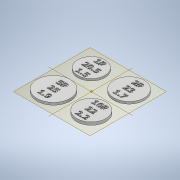
# Autodesk Inventor part: Монеты
Saved by Autodesk Inventor 2020 (Build 240168000, 168)
## iProperties
Created: 2019-12-21
Part Number: Монеты
Material: Типовые
Document SubType Name: Modeling
Designer: Css38
Density: 1 g/cm^3
Appearance: По умолчанию
Author: Css38
Autodesk Inventor part; units mm, degrees
ref_plane "YZ Plane" through (0, 0, 0) normal (1, 0, 0) x (0, 1, 0)
ref_plane "XZ Plane" through (0, 0, 0) normal (0, 1, 0) x (-1, 0, 0)
sketch "Эскиз1" plane through (0, 0, 0) normal (0, 0, 1) x (1, 0, 0)
  circle A0 centre (-14.2806, 14.2806) radius 10.25
  circle A1 centre (14.2806, 14.2806) radius 11.5
  circle A2 centre (-14.2806, -14.2806) radius 12.5
  circle A3 centre (14.2806, -14.2806) radius 11
  line L0 (-37.2928, 0) -> (36.2928, 0) construction
  line L1 (-14.2806, -14.2806) -> (-14.2806, 0) construction
  line L2 (-14.2806, -14.2806) -> (0, -14.2806) construction
  line L3 (14.2806, -14.2806) -> (0, -14.2806) construction
  line L4 (14.2806, -14.2806) -> (14.2806, 0) construction
  line L5 (14.2806, 14.2806) -> (14.2806, 0) construction
  line L6 (14.2806, 14.2806) -> (0, 14.2806) construction
  line L7 (0, 14.2806) -> (-14.2806, 14.2806) construction
  line L8 (-14.2806, 14.2806) -> (-14.2806, 0) construction
  line L9 (0, -37.2928) -> (0, 36.2928) construction
  point P0 (0, 0)
  dimension "d0" = 20.5
  dimension "d1" = 23
  dimension "d2" = 25
  dimension "d3" = 22
  constraints: 16 end point, 8 perpendicular, 4 centre point, 3 point on line, 2 collinear, 2 horizontal, 2 horizontal alignment, 2 vertical alignment
  measures "d0" diameter of A0
  measures "d1" diameter of A1
  measures "d2" diameter of A2
  measures "d3" diameter of A3
extrude "Выдавливание1" add sketch "Эскиз1" along normal blind 1.5 contours A0
extrude "Выдавливание2" add sketch "Эскиз1" along normal blind 1.7 contours A1
extrude "Выдавливание3" add sketch "Эскиз1" along normal blind 1.8 contours A2
extrude "Выдавливание4" add sketch "Эскиз1" along normal blind 2.2 contours A3
sketch "Эскиз2" plane through (-14.2806, 14.2806, 1.5) normal (0, 0, 1) x (1, 0, 0)
  line L0 (-10.25, 10.25) -> (10.25, 10.25) construction
  line L1 (10.25, 10.25) -> (10.25, -10.25) construction
  line L2 (10.25, -10.25) -> (-10.25, -10.25) construction
  line L3 (-10.25, -10.25) -> (-10.25, 10.25) construction
  circle A0 centre (0, 0) radius 10.25 construction
  line L4 (-0.3371, 4.6232) -> (-2.9789, 4.6232)
  line L5 (-2.9789, 4.6232) -> (-2.9789, 5.3201)
  line L6 (-2.9789, 5.3201) -> (-2.1361, 5.3201)
  line L7 (-2.1361, 5.3201) -> (-2.1361, 7.4368)
  line L8 (-2.1361, 7.4368) -> (-2.9789, 7.4368)
  line L9 (-2.9789, 7.4368) -> (-2.9789, 8.0883)
  spline S0 degree 2 poles (-2.9789, 8.0883) (-2.7942, 8.0883) (-2.4279, 8.1369) (-2.3177, 8.1888) knots 0 0 0 1 2 2 2
  spline S1 degree 2 poles (-2.3177, 8.1888) (-2.1912, 8.2536) (-2.0486, 8.4708) (-2.0357, 8.6329) knots 0 0 0 1 2 2 2
  line L10 (-2.0357, 8.6329) -> (-1.1605, 8.6329)
  line L11 (-1.1605, 8.6329) -> (-1.1605, 5.3201)
  line L12 (-1.1605, 5.3201) -> (-0.3371, 5.3201)
  line L13 (-0.3371, 5.3201) -> (-0.3371, 4.6232)
  line L14 (2.4084, 5.6929) -> (2.4084, 5.1224)
  line L15 (2.4084, 5.1224) -> (1.3323, 5.1224)
  line L16 (1.3323, 5.1224) -> (1.3323, 4.6232)
  line L17 (1.3323, 4.6232) -> (0.3339, 4.6232)
  line L18 (0.3339, 4.6232) -> (0.3339, 5.1224)
  line L19 (0.3339, 5.1224) -> (0.0583, 5.1224)
  line L20 (0.0583, 5.1224) -> (0.0583, 5.6929)
  line L21 (0.0583, 5.6929) -> (0.3339, 5.6929)
  line L22 (0.3339, 5.6929) -> (0.3339, 6.0916)
  line L23 (0.3339, 6.0916) -> (0.0583, 6.0916)
  line L24 (0.0583, 6.0916) -> (0.0583, 6.8112)
  line L25 (0.0583, 6.8112) -> (0.3339, 6.8112)
  line L26 (0.3339, 6.8112) -> (0.3339, 8.6232)
  line L27 (0.3339, 8.6232) -> (1.8606, 8.6232)
  spline S2 degree 2 poles (1.8606, 8.6232) (2.1783, 8.6232) (2.7358, 8.4903) (3.1475, 8.1921) (3.3841, 7.7123) (3.3841, 7.3655) knots 0 0 0 1 2 3 4 4 4
  spline S3 degree 2 poles (3.3841, 7.3655) (3.3841, 7.0251) (3.141, 6.5421) (2.7229, 6.2342) (2.1588, 6.0916) (1.8379, 6.0916) knots 0 0 0 1 2 3 4 4 4
  line L28 (1.8379, 6.0916) -> (1.3323, 6.0916)
  line L29 (1.3323, 6.0916) -> (1.3323, 5.6929)
  line L30 (1.3323, 5.6929) -> (2.4084, 5.6929)
  spline S4 degree 2 poles (2.3533, 7.3395) (2.3533, 7.534) (2.1815, 7.7512) (1.9157, 7.8614) (1.5981, 7.8874) (1.4522, 7.8874) knots 0 0 0 1 2 3 4 4 4
  line L31 (1.4522, 7.8874) -> (1.3323, 7.8874)
  line L32 (1.3323, 7.8874) -> (1.3323, 6.8112)
  line L33 (1.3323, 6.8112) -> (1.3744, 6.8112)
  spline S5 degree 2 poles (1.3744, 6.8112) (1.5721, 6.8112) (1.9254, 6.8339) (2.1945, 6.9376) (2.3533, 7.1483) (2.3533, 7.3395) knots 0 0 0 1 2 3 4 4 4
  line L34 (-2.7699, -1.9627) -> (-5.7099, -1.9627)
  line L35 (-5.7099, -1.9627) -> (-5.7099, -1.3112)
  spline S6 degree 2 poles (-5.7099, -1.3112) (-5.3371, -1.013) (-4.7407, -0.4878) (-4.517, -0.2512) knots 0 0 0 1 2 2 2
  spline S7 degree 2 poles (-4.517, -0.2512) (-4.222, 0.0567) (-3.9595, 0.5267) (-3.9595, 0.7731) knots 0 0 0 1 2 2 2
  spline S8 degree 2 poles (-3.9595, 0.7731) (-3.9595, 1.0519) (-4.2934, 1.3501) (-4.5916, 1.3501) knots 0 0 0 1 2 2 2
  spline S9 degree 2 poles (-4.5916, 1.3501) (-4.7439, 1.3501) (-5.0162, 1.2755) (-5.1556, 1.2172) knots 0 0 0 1 2 2 2
  spline S10 degree 2 poles (-5.1556, 1.2172) (-5.2917, 1.1556) (-5.4862, 1.0259) (-5.5348, 0.9935) knots 0 0 0 1 2 2 2
  line L36 (-5.5348, 0.9935) -> (-5.6126, 0.9935)
  line L37 (-5.6126, 0.9935) -> (-5.6126, 1.8655)
  spline S11 degree 2 poles (-5.6126, 1.8655) (-5.4441, 1.9465) (-4.7245, 2.1151) (-4.3906, 2.1151) knots 0 0 0 1 2 2 2
  spline S12 degree 2 poles (-4.3906, 2.1151) (-3.6775, 2.1151) (-2.9449, 1.4797) (-2.9449, 0.906) knots 0 0 0 1 2 2 2
  spline S13 degree 2 poles (-2.9449, 0.906) (-2.9449, 0.5527) (-3.2788, -0.128) (-3.6645, -0.517) knots 0 0 0 1 2 2 2
  spline S14 degree 2 poles (-3.6645, -0.517) (-3.9076, -0.7569) (-4.3647, -1.1297) (-4.4652, -1.2075) knots 0 0 0 1 2 2 2
  line L38 (-4.4652, -1.2075) -> (-2.7699, -1.2075)
  line L39 (-2.7699, -1.2075) -> (-2.7699, -1.9627)
  spline S15 degree 2 poles (0.6823, 0.0373) (0.6823, -0.4814) (0.517, -1.2593) (0.3323, -1.5219) knots 0 0 0 1 2 2 2
  spline S16 degree 2 poles (0.3323, -1.5219) (0.1507, -1.7812) (-0.436, -2.047) (-0.8574, -2.047) knots 0 0 0 1 2 2 2
  spline S17 degree 2 poles (-0.8574, -2.047) (-1.282, -2.047) (-1.8655, -1.7812) (-2.0502, -1.5154) knots 0 0 0 1 2 2 2
  spline S18 degree 2 poles (-2.0502, -1.5154) (-2.235, -1.2528) (-2.4003, -0.4814) (-2.4003, 0.0373) knots 0 0 0 1 2 2 2
  spline S19 degree 2 poles (-2.4003, 0.0373) (-2.4003, 0.5689) (-2.235, 1.3209) (-2.047, 1.5932) knots 0 0 0 1 2 2 2
  spline S20 degree 2 poles (-2.047, 1.5932) (-1.859, 1.859) (-1.2658, 2.1183) (-0.8574, 2.1183) knots 0 0 0 1 2 2 2
  spline S21 degree 2 poles (-0.8574, 2.1183) (-0.4263, 2.1183) (0.1507, 1.846) (0.3355, 1.577) knots 0 0 0 1 2 2 2
  spline S22 degree 2 poles (0.3355, 1.577) (0.517, 1.3144) (0.6823, 0.5397) (0.6823, 0.0373) knots 0 0 0 1 2 2 2
  spline S23 degree 2 poles (-0.3258, 0.0373) (-0.3258, 0.7796) (-0.5689, 1.3793) (-0.8574, 1.3793) knots 0 0 0 1 2 2 2
  spline S24 degree 2 poles (-0.8574, 1.3793) (-1.1459, 1.3793) (-1.3922, 0.7796) (-1.3922, 0.034) knots 0 0 0 1 2 2 2
  spline S25 degree 2 poles (-1.3922, 0.034) (-1.3922, -0.6985) (-1.1459, -1.3079) (-0.8574, -1.3079) knots 0 0 0 1 2 2 2
  spline S26 degree 2 poles (-0.8574, -1.3079) (-0.5721, -1.3079) (-0.3258, -0.6985) (-0.3258, 0.0373) knots 0 0 0 1 2 2 2
  line L40 (2.2253, -1.9627) -> (1.2755, -1.9627)
  line L41 (1.2755, -1.9627) -> (1.2755, -0.906)
  line L42 (1.2755, -0.906) -> (2.2253, -0.906)
  line L43 (2.2253, -0.906) -> (2.2253, -1.9627)
  spline S27 degree 2 poles (5.8655, -0.6078) (5.8655, -0.9222) (5.6515, -1.4538) (5.4408, -1.6451) knots 0 0 0 1 2 2 2
  spline S28 degree 2 poles (5.4408, -1.6451) (5.2301, -1.8363) (4.6532, -2.047) (4.2318, -2.047) knots 0 0 0 1 2 2 2
  spline S29 degree 2 poles (4.2318, -2.047) (3.7844, -2.0438) (3.1426, -1.8979) (2.9319, -1.8039) knots 0 0 0 1 2 2 2
  line L44 (2.9319, -1.8039) -> (2.9319, -0.9319)
  line L45 (2.9319, -0.9319) -> (3.0227, -0.9319)
  spline S30 degree 2 poles (3.0227, -0.9319) (3.1005, -0.9741) (3.2885, -1.0843) (3.4408, -1.1426) knots 0 0 0 1 2 2 2
  spline S31 degree 2 poles (3.4408, -1.1426) (3.5835, -1.1977) (3.8784, -1.2723) (4.0567, -1.2723) knots 0 0 0 1 2 2 2
  spline S32 degree 2 poles (4.0567, -1.2723) (4.2123, -1.2723) (4.5754, -1.1945) (4.6856, -1.0908) knots 0 0 0 1 2 2 2
  spline S33 degree 2 poles (4.6856, -1.0908) (4.7666, -1.0097) (4.8574, -0.812) (4.8574, -0.6467) knots 0 0 0 1 2 2 2
  spline S34 degree 2 poles (4.8574, -0.6467) (4.8574, -0.5041) (4.7407, -0.3031) (4.6467, -0.2415) knots 0 0 0 1 2 2 2
  spline S35 degree 2 poles (4.6467, -0.2415) (4.5105, -0.1507) (4.1216, -0.0989) (3.9822, -0.0989) knots 0 0 0 1 2 2 2
  spline S36 degree 2 poles (3.9822, -0.0989) (3.7618, -0.0989) (3.3436, -0.1702) (3.1912, -0.2091) knots 0 0 0 1 2 2 2
  line L46 (3.1912, -0.2091) -> (3.1037, -0.2091)
  line L47 (3.1037, -0.2091) -> (3.1037, 2.0373)
  line L48 (3.1037, 2.0373) -> (5.7553, 2.0373)
  line L49 (5.7553, 2.0373) -> (5.7553, 1.282)
  line L50 (5.7553, 1.282) -> (4.0535, 1.282)
  line L51 (4.0535, 1.282) -> (4.0535, 0.6175)
  spline S37 degree 2 poles (4.0535, 0.6175) (4.1345, 0.624) (4.3582, 0.6305) (4.4198, 0.6305) knots 0 0 0 1 2 2 2
  spline S38 degree 2 poles (4.4198, 0.6305) (4.7083, 0.6305) (5.1945, 0.5138) (5.3857, 0.3938) knots 0 0 0 1 2 2 2
  spline S39 degree 2 poles (5.3857, 0.3938) (5.6126, 0.2447) (5.8655, -0.2512) (5.8655, -0.6078) knots 0 0 0 1 2 2 2
  line L52 (-1.1961, -8.5486) -> (-3.8379, -8.5486)
  line L53 (-3.8379, -8.5486) -> (-3.8379, -7.8517)
  line L54 (-3.8379, -7.8517) -> (-2.9951, -7.8517)
  line L55 (-2.9951, -7.8517) -> (-2.9951, -5.735)
  line L56 (-2.9951, -5.735) -> (-3.8379, -5.735)
  line L57 (-3.8379, -5.735) -> (-3.8379, -5.0835)
  spline S40 degree 2 poles (-3.8379, -5.0835) (-3.6532, -5.0835) (-3.2869, -5.0348) (-3.1767, -4.983) knots 0 0 0 1 2 2 2
  spline S41 degree 2 poles (-3.1767, -4.983) (-3.0502, -4.9181) (-2.9076, -4.701) (-2.8947, -4.5389) knots 0 0 0 1 2 2 2
  line L58 (-2.8947, -4.5389) -> (-2.0194, -4.5389)
  line L59 (-2.0194, -4.5389) -> (-2.0194, -7.8517)
  line L60 (-2.0194, -7.8517) -> (-1.1961, -7.8517)
  line L61 (-1.1961, -7.8517) -> (-1.1961, -8.5486)
  line L62 (0.4733, -8.5486) -> (-0.4765, -8.5486)
  line L63 (-0.4765, -8.5486) -> (-0.4765, -7.4919)
  line L64 (-0.4765, -7.4919) -> (0.4733, -7.4919)
  line L65 (0.4733, -7.4919) -> (0.4733, -8.5486)
  spline S42 degree 2 poles (4.1135, -7.1937) (4.1135, -7.5081) (3.8995, -8.0397) (3.6888, -8.231) knots 0 0 0 1 2 2 2
  spline S43 degree 2 poles (3.6888, -8.231) (3.4781, -8.4222) (2.9011, -8.6329) (2.4797, -8.6329) knots 0 0 0 1 2 2 2
  spline S44 degree 2 poles (2.4797, -8.6329) (2.0324, -8.6297) (1.3906, -8.4838) (1.1799, -8.3898) knots 0 0 0 1 2 2 2
  line L66 (1.1799, -8.3898) -> (1.1799, -7.5178)
  line L67 (1.1799, -7.5178) -> (1.2707, -7.5178)
  spline S45 degree 2 poles (1.2707, -7.5178) (1.3485, -7.56) (1.5365, -7.6702) (1.6888, -7.7285) knots 0 0 0 1 2 2 2
  spline S46 degree 2 poles (1.6888, -7.7285) (1.8314, -7.7836) (2.1264, -7.8582) (2.3047, -7.8582) knots 0 0 0 1 2 2 2
  spline S47 degree 2 poles (2.3047, -7.8582) (2.4603, -7.8582) (2.8233, -7.7804) (2.9335, -7.6767) knots 0 0 0 1 2 2 2
  spline S48 degree 2 poles (2.9335, -7.6767) (3.0146, -7.5956) (3.1053, -7.3979) (3.1053, -7.2326) knots 0 0 0 1 2 2 2
  spline S49 degree 2 poles (3.1053, -7.2326) (3.1053, -7.0899) (2.9887, -6.889) (2.8947, -6.8274) knots 0 0 0 1 2 2 2
  spline S50 degree 2 poles (2.8947, -6.8274) (2.7585, -6.7366) (2.3695, -6.6848) (2.2301, -6.6848) knots 0 0 0 1 2 2 2
  spline S51 degree 2 poles (2.2301, -6.6848) (2.0097, -6.6848) (1.5916, -6.7561) (1.4392, -6.795) knots 0 0 0 1 2 2 2
  line L68 (1.4392, -6.795) -> (1.3517, -6.795)
  line L69 (1.3517, -6.795) -> (1.3517, -4.5486)
  line L70 (1.3517, -4.5486) -> (4.0032, -4.5486)
  line L71 (4.0032, -4.5486) -> (4.0032, -5.3039)
  line L72 (4.0032, -5.3039) -> (2.3015, -5.3039)
  line L73 (2.3015, -5.3039) -> (2.3015, -5.9684)
  spline S52 degree 2 poles (2.3015, -5.9684) (2.3825, -5.9619) (2.6062, -5.9554) (2.6677, -5.9554) knots 0 0 0 1 2 2 2
  spline S53 degree 2 poles (2.6677, -5.9554) (2.9562, -5.9554) (3.4425, -6.0721) (3.6337, -6.1921) knots 0 0 0 1 2 2 2
  spline S54 degree 2 poles (3.6337, -6.1921) (3.8606, -6.3412) (4.1135, -6.8371) (4.1135, -7.1937) knots 0 0 0 1 2 2 2
  point P0 (10.25, 0)
  point P1 (-10.25, 0)
  point P2 (0, 10.25)
  point P3 (0, -10.25)
  constraints: 4 midpoint, 4 point on circle, 2 other
emboss "Рельеф5" sketch "Эскиз2" operation cut depth 0.5 direction (0, 0, -1)
sketch "Эскиз3" plane through (14.2806, 14.2806, 1.7) normal (0, 0, 1) x (1, 0, 0)
  line L0 (-11.5, 11.5) -> (11.5, 11.5) construction
  line L1 (11.5, 11.5) -> (11.5, -11.5) construction
  line L2 (11.5, -11.5) -> (-11.5, -11.5) construction
  line L3 (-11.5, -11.5) -> (-11.5, 11.5) construction
  circle A0 centre (0, 0) radius 11.5 construction
  line L4 (-0.1588, 4.547) -> (-3.0989, 4.547)
  line L5 (-3.0989, 4.547) -> (-3.0989, 5.1985)
  spline S0 degree 2 poles (-3.0989, 5.1985) (-2.7261, 5.4968) (-2.1297, 6.0219) (-1.906, 6.2585) knots 0 0 0 1 2 2 2
  spline S1 degree 2 poles (-1.906, 6.2585) (-1.611, 6.5664) (-1.3485, 7.0365) (-1.3485, 7.2828) knots 0 0 0 1 2 2 2
  spline S2 degree 2 poles (-1.3485, 7.2828) (-1.3485, 7.5616) (-1.6823, 7.8598) (-1.9806, 7.8598) knots 0 0 0 1 2 2 2
  spline S3 degree 2 poles (-1.9806, 7.8598) (-2.1329, 7.8598) (-2.4052, 7.7852) (-2.5446, 7.7269) knots 0 0 0 1 2 2 2
  spline S4 degree 2 poles (-2.5446, 7.7269) (-2.6807, 7.6653) (-2.8752, 7.5357) (-2.9238, 7.5032) knots 0 0 0 1 2 2 2
  line L6 (-2.9238, 7.5032) -> (-3.0016, 7.5032)
  line L7 (-3.0016, 7.5032) -> (-3.0016, 8.3752)
  spline S5 degree 2 poles (-3.0016, 8.3752) (-2.8331, 8.4562) (-2.1135, 8.6248) (-1.7796, 8.6248) knots 0 0 0 1 2 2 2
  spline S6 degree 2 poles (-1.7796, 8.6248) (-1.0665, 8.6248) (-0.3339, 7.9895) (-0.3339, 7.4157) knots 0 0 0 1 2 2 2
  spline S7 degree 2 poles (-0.3339, 7.4157) (-0.3339, 7.0624) (-0.6677, 6.3817) (-1.0535, 5.9927) knots 0 0 0 1 2 2 2
  spline S8 degree 2 poles (-1.0535, 5.9927) (-1.2966, 5.7528) (-1.7536, 5.3801) (-1.8541, 5.3023) knots 0 0 0 1 2 2 2
  line L8 (-1.8541, 5.3023) -> (-0.1588, 5.3023)
  line L9 (-0.1588, 5.3023) -> (-0.1588, 4.547)
  line L10 (2.4084, 5.6167) -> (2.4084, 5.0462)
  line L11 (2.4084, 5.0462) -> (1.3323, 5.0462)
  line L12 (1.3323, 5.0462) -> (1.3323, 4.547)
  line L13 (1.3323, 4.547) -> (0.3339, 4.547)
  line L14 (0.3339, 4.547) -> (0.3339, 5.0462)
  line L15 (0.3339, 5.0462) -> (0.0583, 5.0462)
  line L16 (0.0583, 5.0462) -> (0.0583, 5.6167)
  line L17 (0.0583, 5.6167) -> (0.3339, 5.6167)
  line L18 (0.3339, 5.6167) -> (0.3339, 6.0154)
  line L19 (0.3339, 6.0154) -> (0.0583, 6.0154)
  line L20 (0.0583, 6.0154) -> (0.0583, 6.735)
  line L21 (0.0583, 6.735) -> (0.3339, 6.735)
  line L22 (0.3339, 6.735) -> (0.3339, 8.547)
  line L23 (0.3339, 8.547) -> (1.8606, 8.547)
  spline S9 degree 2 poles (1.8606, 8.547) (2.1783, 8.547) (2.7358, 8.4141) (3.1475, 8.1159) (3.3841, 7.6361) (3.3841, 7.2893) knots 0 0 0 1 2 3 4 4 4
  spline S10 degree 2 poles (3.3841, 7.2893) (3.3841, 6.9489) (3.141, 6.466) (2.7229, 6.158) (2.1588, 6.0154) (1.8379, 6.0154) knots 0 0 0 1 2 3 4 4 4
  line L24 (1.8379, 6.0154) -> (1.3323, 6.0154)
  line L25 (1.3323, 6.0154) -> (1.3323, 5.6167)
  line L26 (1.3323, 5.6167) -> (2.4084, 5.6167)
  spline S11 degree 2 poles (2.3533, 7.2634) (2.3533, 7.4579) (2.1815, 7.675) (1.9157, 7.7852) (1.5981, 7.8112) (1.4522, 7.8112) knots 0 0 0 1 2 3 4 4 4
  line L27 (1.4522, 7.8112) -> (1.3323, 7.8112)
  line L28 (1.3323, 7.8112) -> (1.3323, 6.735)
  line L29 (1.3323, 6.735) -> (1.3744, 6.735)
  spline S12 degree 2 poles (1.3744, 6.735) (1.5721, 6.735) (1.9254, 6.7577) (2.1945, 6.8614) (2.3533, 7.0721) (2.3533, 7.2634) knots 0 0 0 1 2 3 4 4 4
  line L30 (-0.1588, -2.0389) -> (-3.0989, -2.0389)
  line L31 (-3.0989, -2.0389) -> (-3.0989, -1.3874)
  spline S13 degree 2 poles (-3.0989, -1.3874) (-2.7261, -1.0891) (-2.1297, -0.564) (-1.906, -0.3274) knots 0 0 0 1 2 2 2
  spline S14 degree 2 poles (-1.906, -0.3274) (-1.611, -0.0194) (-1.3485, 0.4506) (-1.3485, 0.6969) knots 0 0 0 1 2 2 2
  spline S15 degree 2 poles (-1.3485, 0.6969) (-1.3485, 0.9757) (-1.6823, 1.2739) (-1.9806, 1.2739) knots 0 0 0 1 2 2 2
  spline S16 degree 2 poles (-1.9806, 1.2739) (-2.1329, 1.2739) (-2.4052, 1.1994) (-2.5446, 1.141) knots 0 0 0 1 2 2 2
  spline S17 degree 2 poles (-2.5446, 1.141) (-2.6807, 1.0794) (-2.8752, 0.9498) (-2.9238, 0.9173) knots 0 0 0 1 2 2 2
  line L32 (-2.9238, 0.9173) -> (-3.0016, 0.9173)
  line L33 (-3.0016, 0.9173) -> (-3.0016, 1.7893)
  spline S18 degree 2 poles (-3.0016, 1.7893) (-2.8331, 1.8703) (-2.1135, 2.0389) (-1.7796, 2.0389) knots 0 0 0 1 2 2 2
  spline S19 degree 2 poles (-1.7796, 2.0389) (-1.0665, 2.0389) (-0.3339, 1.4036) (-0.3339, 0.8298) knots 0 0 0 1 2 2 2
  spline S20 degree 2 poles (-0.3339, 0.8298) (-0.3339, 0.4765) (-0.6677, -0.2042) (-1.0535, -0.5932) knots 0 0 0 1 2 2 2
  spline S21 degree 2 poles (-1.0535, -0.5932) (-1.2966, -0.8331) (-1.7536, -1.2058) (-1.8541, -1.2836) knots 0 0 0 1 2 2 2
  line L34 (-1.8541, -1.2836) -> (-0.1588, -1.2836)
  line L35 (-0.1588, -1.2836) -> (-0.1588, -2.0389)
  spline S22 degree 2 poles (3.2447, -0.8266) (3.2447, -1.1216) (3.0276, -1.6045) (2.8169, -1.7731) knots 0 0 0 1 2 2 2
  spline S23 degree 2 poles (2.8169, -1.7731) (2.6062, -1.9417) (2.0324, -2.1232) (1.6207, -2.1232) knots 0 0 0 1 2 2 2
  spline S24 degree 2 poles (1.6207, -2.1232) (1.154, -2.1232) (0.4862, -1.9676) (0.2755, -1.8703) knots 0 0 0 1 2 2 2
  line L36 (0.2755, -1.8703) -> (0.2755, -1.0016)
  line L37 (0.2755, -1.0016) -> (0.3728, -1.0016)
  spline S25 degree 2 poles (0.3728, -1.0016) (0.5932, -1.141) (1.1864, -1.3485) (1.4327, -1.3485) knots 0 0 0 1 2 2 2
  spline S26 degree 2 poles (1.4327, -1.3485) (1.5786, -1.3485) (1.919, -1.2966) (2.0357, -1.2123) knots 0 0 0 1 2 2 2
  spline S27 degree 2 poles (2.0357, -1.2123) (2.1264, -1.1442) (2.2366, -0.9465) (2.2366, -0.7682) knots 0 0 0 1 2 2 2
  spline S28 degree 2 poles (2.2366, -0.7682) (2.2366, -0.59) (2.081, -0.3987) (1.9514, -0.3533) knots 0 0 0 1 2 2 2
  spline S29 degree 2 poles (1.9514, -0.3533) (1.8217, -0.3079) (1.4619, -0.2982) (1.3225, -0.2982) knots 0 0 0 1 2 2 2
  line L38 (1.3225, -0.2982) -> (1.1507, -0.2982)
  line L39 (1.1507, -0.2982) -> (1.1507, 0.4052)
  line L40 (1.1507, 0.4052) -> (1.3096, 0.4052)
  spline S30 degree 2 poles (1.3096, 0.4052) (1.4911, 0.4052) (1.799, 0.4376) (1.906, 0.4862) knots 0 0 0 1 2 2 2
  spline S31 degree 2 poles (1.906, 0.4862) (2.013, 0.5381) (2.1329, 0.7196) (2.1329, 0.8752) knots 0 0 0 1 2 2 2
  spline S32 degree 2 poles (2.1329, 0.8752) (2.1329, 0.9984) (2.0194, 1.1507) (1.9384, 1.1929) knots 0 0 0 1 2 2 2
  spline S33 degree 2 poles (1.9384, 1.1929) (1.8412, 1.2415) (1.5818, 1.2739) (1.4911, 1.2739) knots 0 0 0 1 2 2 2
  spline S34 degree 2 poles (1.4911, 1.2739) (1.3452, 1.2739) (1.0373, 1.2058) (0.8947, 1.1507) knots 0 0 0 1 2 2 2
  spline S35 degree 2 poles (0.8947, 1.1507) (0.7812, 1.1086) (0.5348, 0.9724) (0.4765, 0.9368) knots 0 0 0 1 2 2 2
  line L41 (0.4765, 0.9368) -> (0.3922, 0.9368)
  line L42 (0.3922, 0.9368) -> (0.3922, 1.7925)
  spline S36 degree 2 poles (0.3922, 1.7925) (0.5997, 1.8801) (1.2998, 2.0454) (1.6661, 2.0454) knots 0 0 0 1 2 2 2
  spline S37 degree 2 poles (1.6661, 2.0454) (2.0227, 2.0454) (2.5478, 1.9222) (2.7326, 1.8023) knots 0 0 0 1 2 2 2
  spline S38 degree 2 poles (2.7326, 1.8023) (2.9368, 1.6759) (3.141, 1.2869) (3.141, 1.0438) knots 0 0 0 1 2 2 2
  spline S39 degree 2 poles (3.141, 1.0438) (3.141, 0.7002) (2.7455, 0.188) (2.4214, 0.1135) knots 0 0 0 1 2 2 2
  line L43 (2.4214, 0.1135) -> (2.4214, 0.0746)
  spline S40 degree 2 poles (2.4214, 0.0746) (2.564, 0.0551) (2.8363, -0.0486) (2.966, -0.1653) knots 0 0 0 1 2 2 2
  spline S41 degree 2 poles (2.966, -0.1653) (3.0859, -0.269) (3.2447, -0.5997) (3.2447, -0.8266) knots 0 0 0 1 2 2 2
  line L44 (-1.1961, -8.6248) -> (-3.8379, -8.6248)
  line L45 (-3.8379, -8.6248) -> (-3.8379, -7.9279)
  line L46 (-3.8379, -7.9279) -> (-2.9951, -7.9279)
  line L47 (-2.9951, -7.9279) -> (-2.9951, -5.8112)
  line L48 (-2.9951, -5.8112) -> (-3.8379, -5.8112)
  line L49 (-3.8379, -5.8112) -> (-3.8379, -5.1596)
  spline S42 degree 2 poles (-3.8379, -5.1596) (-3.6532, -5.1596) (-3.2869, -5.111) (-3.1767, -5.0592) knots 0 0 0 1 2 2 2
  spline S43 degree 2 poles (-3.1767, -5.0592) (-3.0502, -4.9943) (-2.9076, -4.7771) (-2.8947, -4.6151) knots 0 0 0 1 2 2 2
  line L50 (-2.8947, -4.6151) -> (-2.0194, -4.6151)
  line L51 (-2.0194, -4.6151) -> (-2.0194, -7.9279)
  line L52 (-2.0194, -7.9279) -> (-1.1961, -7.9279)
  line L53 (-1.1961, -7.9279) -> (-1.1961, -8.6248)
  line L54 (0.4733, -8.6248) -> (-0.4765, -8.6248)
  line L55 (-0.4765, -8.6248) -> (-0.4765, -7.5681)
  line L56 (-0.4765, -7.5681) -> (0.4733, -7.5681)
  line L57 (0.4733, -7.5681) -> (0.4733, -8.6248)
  line L58 (4.1167, -5.419) -> (2.4084, -8.6248)
  line L59 (2.4084, -8.6248) -> (1.2934, -8.6248)
  line L60 (1.2934, -8.6248) -> (3.0794, -5.3801)
  line L61 (3.0794, -5.3801) -> (1.1734, -5.3801)
  line L62 (1.1734, -5.3801) -> (1.1734, -4.6248)
  line L63 (1.1734, -4.6248) -> (4.1167, -4.6248)
  line L64 (4.1167, -4.6248) -> (4.1167, -5.419)
  point P0 (0, 11.5)
  point P1 (11.5, 0)
  point P2 (0, -11.5)
  point P3 (-11.5, 0)
  constraints: 4 midpoint, 4 point on circle, 2 other
emboss "Рельеф6" sketch "Эскиз3" operation cut depth 0.5 direction (0, 0, -1)
sketch "Эскиз4" plane through (-14.2806, -14.2806, 1.8) normal (0, 0, 1) x (1, 0, 0)
  line L0 (-12.5, 12.5) -> (12.5, 12.5) construction
  line L1 (12.5, 12.5) -> (12.5, -12.5) construction
  line L2 (12.5, -12.5) -> (-12.5, -12.5) construction
  line L3 (-12.5, -12.5) -> (-12.5, 12.5) construction
  circle A0 centre (0, 0) radius 12.5 construction
  spline S0 degree 2 poles (-0.2496, 5.9797) (-0.2496, 5.6653) (-0.4635, 5.1337) (-0.6742, 4.9425) knots 0 0 0 1 2 2 2
  spline S1 degree 2 poles (-0.6742, 4.9425) (-0.8849, 4.7512) (-1.4619, 4.5405) (-1.8833, 4.5405) knots 0 0 0 1 2 2 2
  spline S2 degree 2 poles (-1.8833, 4.5405) (-2.3306, 4.5438) (-2.9724, 4.6896) (-3.1831, 4.7836) knots 0 0 0 1 2 2 2
  line L4 (-3.1831, 4.7836) -> (-3.1831, 5.6556)
  line L5 (-3.1831, 5.6556) -> (-3.0924, 5.6556)
  spline S3 degree 2 poles (-3.0924, 5.6556) (-3.0146, 5.6134) (-2.8266, 5.5032) (-2.6742, 5.4449) knots 0 0 0 1 2 2 2
  spline S4 degree 2 poles (-2.6742, 5.4449) (-2.5316, 5.3898) (-2.2366, 5.3152) (-2.0583, 5.3152) knots 0 0 0 1 2 2 2
  spline S5 degree 2 poles (-2.0583, 5.3152) (-1.9028, 5.3152) (-1.5397, 5.393) (-1.4295, 5.4968) knots 0 0 0 1 2 2 2
  spline S6 degree 2 poles (-1.4295, 5.4968) (-1.3485, 5.5778) (-1.2577, 5.7755) (-1.2577, 5.9408) knots 0 0 0 1 2 2 2
  spline S7 degree 2 poles (-1.2577, 5.9408) (-1.2577, 6.0835) (-1.3744, 6.2844) (-1.4684, 6.346) knots 0 0 0 1 2 2 2
  spline S8 degree 2 poles (-1.4684, 6.346) (-1.6045, 6.4368) (-1.9935, 6.4886) (-2.1329, 6.4886) knots 0 0 0 1 2 2 2
  spline S9 degree 2 poles (-2.1329, 6.4886) (-2.3533, 6.4886) (-2.7715, 6.4173) (-2.9238, 6.3784) knots 0 0 0 1 2 2 2
  line L6 (-2.9238, 6.3784) -> (-3.0113, 6.3784)
  line L7 (-3.0113, 6.3784) -> (-3.0113, 8.6248)
  line L8 (-3.0113, 8.6248) -> (-0.3598, 8.6248)
  line L9 (-0.3598, 8.6248) -> (-0.3598, 7.8695)
  line L10 (-0.3598, 7.8695) -> (-2.0616, 7.8695)
  line L11 (-2.0616, 7.8695) -> (-2.0616, 7.205)
  spline S10 degree 2 poles (-2.0616, 7.205) (-1.9806, 7.2115) (-1.7569, 7.218) (-1.6953, 7.218) knots 0 0 0 1 2 2 2
  spline S11 degree 2 poles (-1.6953, 7.218) (-1.4068, 7.218) (-0.9206, 7.1013) (-0.7293, 6.9814) knots 0 0 0 1 2 2 2
  spline S12 degree 2 poles (-0.7293, 6.9814) (-0.5024, 6.8322) (-0.2496, 6.3363) (-0.2496, 5.9797) knots 0 0 0 1 2 2 2
  line L12 (2.4084, 5.6945) -> (2.4084, 5.124)
  line L13 (2.4084, 5.124) -> (1.3323, 5.124)
  line L14 (1.3323, 5.124) -> (1.3323, 4.6248)
  line L15 (1.3323, 4.6248) -> (0.3339, 4.6248)
  line L16 (0.3339, 4.6248) -> (0.3339, 5.124)
  line L17 (0.3339, 5.124) -> (0.0583, 5.124)
  line L18 (0.0583, 5.124) -> (0.0583, 5.6945)
  line L19 (0.0583, 5.6945) -> (0.3339, 5.6945)
  line L20 (0.3339, 5.6945) -> (0.3339, 6.0932)
  line L21 (0.3339, 6.0932) -> (0.0583, 6.0932)
  line L22 (0.0583, 6.0932) -> (0.0583, 6.8128)
  line L23 (0.0583, 6.8128) -> (0.3339, 6.8128)
  line L24 (0.3339, 6.8128) -> (0.3339, 8.6248)
  line L25 (0.3339, 8.6248) -> (1.8606, 8.6248)
  spline S13 degree 2 poles (1.8606, 8.6248) (2.1783, 8.6248) (2.7358, 8.4919) (3.1475, 8.1937) (3.3841, 7.7139) (3.3841, 7.3671) knots 0 0 0 1 2 3 4 4 4
  spline S14 degree 2 poles (3.3841, 7.3671) (3.3841, 7.0267) (3.141, 6.5438) (2.7229, 6.2358) (2.1588, 6.0932) (1.8379, 6.0932) knots 0 0 0 1 2 3 4 4 4
  line L26 (1.8379, 6.0932) -> (1.3323, 6.0932)
  line L27 (1.3323, 6.0932) -> (1.3323, 5.6945)
  line L28 (1.3323, 5.6945) -> (2.4084, 5.6945)
  spline S15 degree 2 poles (2.3533, 7.3412) (2.3533, 7.5357) (2.1815, 7.7528) (1.9157, 7.863) (1.5981, 7.889) (1.4522, 7.889) knots 0 0 0 1 2 3 4 4 4
  line L29 (1.4522, 7.889) -> (1.3323, 7.889)
  line L30 (1.3323, 7.889) -> (1.3323, 6.8128)
  line L31 (1.3323, 6.8128) -> (1.3744, 6.8128)
  spline S16 degree 2 poles (1.3744, 6.8128) (1.5721, 6.8128) (1.9254, 6.8355) (2.1945, 6.9392) (2.3533, 7.1499) (2.3533, 7.3412) knots 0 0 0 1 2 3 4 4 4
  line L32 (-0.1588, -1.9611) -> (-3.0989, -1.9611)
  line L33 (-3.0989, -1.9611) -> (-3.0989, -1.3096)
  spline S17 degree 2 poles (-3.0989, -1.3096) (-2.7261, -1.0113) (-2.1297, -0.4862) (-1.906, -0.2496) knots 0 0 0 1 2 2 2
  spline S18 degree 2 poles (-1.906, -0.2496) (-1.611, 0.0583) (-1.3485, 0.5284) (-1.3485, 0.7747) knots 0 0 0 1 2 2 2
  spline S19 degree 2 poles (-1.3485, 0.7747) (-1.3485, 1.0535) (-1.6823, 1.3517) (-1.9806, 1.3517) knots 0 0 0 1 2 2 2
  spline S20 degree 2 poles (-1.9806, 1.3517) (-2.1329, 1.3517) (-2.4052, 1.2771) (-2.5446, 1.2188) knots 0 0 0 1 2 2 2
  spline S21 degree 2 poles (-2.5446, 1.2188) (-2.6807, 1.1572) (-2.8752, 1.0276) (-2.9238, 0.9951) knots 0 0 0 1 2 2 2
  line L34 (-2.9238, 0.9951) -> (-3.0016, 0.9951)
  line L35 (-3.0016, 0.9951) -> (-3.0016, 1.8671)
  spline S22 degree 2 poles (-3.0016, 1.8671) (-2.8331, 1.9481) (-2.1135, 2.1167) (-1.7796, 2.1167) knots 0 0 0 1 2 2 2
  spline S23 degree 2 poles (-1.7796, 2.1167) (-1.0665, 2.1167) (-0.3339, 1.4814) (-0.3339, 0.9076) knots 0 0 0 1 2 2 2
  spline S24 degree 2 poles (-0.3339, 0.9076) (-0.3339, 0.5543) (-0.6677, -0.1264) (-1.0535, -0.5154) knots 0 0 0 1 2 2 2
  spline S25 degree 2 poles (-1.0535, -0.5154) (-1.2966, -0.7553) (-1.7536, -1.128) (-1.8541, -1.2058) knots 0 0 0 1 2 2 2
  line L36 (-1.8541, -1.2058) -> (-0.1588, -1.2058)
  line L37 (-0.1588, -1.2058) -> (-0.1588, -1.9611)
  spline S26 degree 2 poles (3.2545, -0.6062) (3.2545, -0.9206) (3.0405, -1.4522) (2.8298, -1.6434) knots 0 0 0 1 2 2 2
  spline S27 degree 2 poles (2.8298, -1.6434) (2.6191, -1.8347) (2.0421, -2.0454) (1.6207, -2.0454) knots 0 0 0 1 2 2 2
  spline S28 degree 2 poles (1.6207, -2.0454) (1.1734, -2.0421) (0.5316, -1.8963) (0.3209, -1.8023) knots 0 0 0 1 2 2 2
  line L38 (0.3209, -1.8023) -> (0.3209, -0.9303)
  line L39 (0.3209, -0.9303) -> (0.4117, -0.9303)
  spline S29 degree 2 poles (0.4117, -0.9303) (0.4895, -0.9724) (0.6775, -1.0827) (0.8298, -1.141) knots 0 0 0 1 2 2 2
  spline S30 degree 2 poles (0.8298, -1.141) (0.9724, -1.1961) (1.2674, -1.2707) (1.4457, -1.2707) knots 0 0 0 1 2 2 2
  spline S31 degree 2 poles (1.4457, -1.2707) (1.6013, -1.2707) (1.9643, -1.1929) (2.0746, -1.0891) knots 0 0 0 1 2 2 2
  spline S32 degree 2 poles (2.0746, -1.0891) (2.1556, -1.0081) (2.2464, -0.8104) (2.2464, -0.6451) knots 0 0 0 1 2 2 2
  spline S33 degree 2 poles (2.2464, -0.6451) (2.2464, -0.5024) (2.1297, -0.3015) (2.0357, -0.2399) knots 0 0 0 1 2 2 2
  spline S34 degree 2 poles (2.0357, -0.2399) (1.8995, -0.1491) (1.5105, -0.0972) (1.3712, -0.0972) knots 0 0 0 1 2 2 2
  spline S35 degree 2 poles (1.3712, -0.0972) (1.1507, -0.0972) (0.7326, -0.1686) (0.5802, -0.2075) knots 0 0 0 1 2 2 2
  line L40 (0.5802, -0.2075) -> (0.4927, -0.2075)
  line L41 (0.4927, -0.2075) -> (0.4927, 2.0389)
  line L42 (0.4927, 2.0389) -> (3.1442, 2.0389)
  line L43 (3.1442, 2.0389) -> (3.1442, 1.2836)
  line L44 (3.1442, 1.2836) -> (1.4425, 1.2836)
  line L45 (1.4425, 1.2836) -> (1.4425, 0.6191)
  spline S36 degree 2 poles (1.4425, 0.6191) (1.5235, 0.6256) (1.7472, 0.6321) (1.8088, 0.6321) knots 0 0 0 1 2 2 2
  spline S37 degree 2 poles (1.8088, 0.6321) (2.0972, 0.6321) (2.5835, 0.5154) (2.7747, 0.3955) knots 0 0 0 1 2 2 2
  spline S38 degree 2 poles (2.7747, 0.3955) (3.0016, 0.2464) (3.2545, -0.2496) (3.2545, -0.6062) knots 0 0 0 1 2 2 2
  line L46 (-1.1961, -8.547) -> (-3.8379, -8.547)
  line L47 (-3.8379, -8.547) -> (-3.8379, -7.8501)
  line L48 (-3.8379, -7.8501) -> (-2.9951, -7.8501)
  line L49 (-2.9951, -7.8501) -> (-2.9951, -5.7334)
  line L50 (-2.9951, -5.7334) -> (-3.8379, -5.7334)
  line L51 (-3.8379, -5.7334) -> (-3.8379, -5.0818)
  spline S39 degree 2 poles (-3.8379, -5.0818) (-3.6532, -5.0818) (-3.2869, -5.0332) (-3.1767, -4.9814) knots 0 0 0 1 2 2 2
  spline S40 degree 2 poles (-3.1767, -4.9814) (-3.0502, -4.9165) (-2.9076, -4.6993) (-2.8947, -4.5373) knots 0 0 0 1 2 2 2
  line L52 (-2.8947, -4.5373) -> (-2.0194, -4.5373)
  line L53 (-2.0194, -4.5373) -> (-2.0194, -7.8501)
  line L54 (-2.0194, -7.8501) -> (-1.1961, -7.8501)
  line L55 (-1.1961, -7.8501) -> (-1.1961, -8.547)
  line L56 (0.4733, -8.547) -> (-0.4765, -8.547)
  line L57 (-0.4765, -8.547) -> (-0.4765, -7.4903)
  line L58 (-0.4765, -7.4903) -> (0.4733, -7.4903)
  line L59 (0.4733, -7.4903) -> (0.4733, -8.547)
  spline S41 degree 2 poles (4.1005, -6.3233) (4.1005, -6.8322) (3.8639, -7.6815) (3.6143, -7.9862) knots 0 0 0 1 2 2 2
  spline S42 degree 2 poles (3.6143, -7.9862) (3.3549, -8.2942) (2.59, -8.6248) (2.0324, -8.6248) knots 0 0 0 1 2 2 2
  spline S43 degree 2 poles (2.0324, -8.6248) (1.8444, -8.6248) (1.436, -8.5762) (1.3679, -8.5567) knots 0 0 0 1 2 2 2
  line L60 (1.3679, -8.5567) -> (1.3679, -7.7723)
  line L61 (1.3679, -7.7723) -> (1.4457, -7.7723)
  spline S44 degree 2 poles (1.4457, -7.7723) (1.5203, -7.8112) (1.799, -7.8955) (2.0421, -7.8955) knots 0 0 0 1 2 2 2
  spline S45 degree 2 poles (2.0421, -7.8955) (2.2399, -7.8955) (2.6062, -7.7917) (2.7358, -7.6783) knots 0 0 0 1 2 2 2
  spline S46 degree 2 poles (2.7358, -7.6783) (2.8752, -7.5583) (3.0567, -7.205) (3.0891, -6.9392) knots 0 0 0 1 2 2 2
  spline S47 degree 2 poles (3.0891, -6.9392) (2.8752, -7.0721) (2.5057, -7.2147) (2.2301, -7.2147) knots 0 0 0 1 2 2 2
  spline S48 degree 2 poles (2.2301, -7.2147) (2.0259, -7.2147) (1.6467, -7.1045) (1.4911, -6.9878) knots 0 0 0 1 2 2 2
  spline S49 degree 2 poles (1.4911, -6.9878) (1.2836, -6.829) (1.0405, -6.3201) (1.0405, -5.9181) knots 0 0 0 1 2 2 2
  spline S50 degree 2 poles (1.0405, -5.9181) (1.0405, -5.6037) (1.2545, -5.0754) (1.4489, -4.8809) knots 0 0 0 1 2 2 2
  spline S51 degree 2 poles (1.4489, -4.8809) (1.6434, -4.6864) (2.2075, -4.466) (2.5543, -4.466) knots 0 0 0 1 2 2 2
  spline S52 degree 2 poles (2.5543, -4.466) (2.9044, -4.466) (3.4457, -4.6604) (3.6402, -4.8647) knots 0 0 0 1 2 2 2
  spline S53 degree 2 poles (3.6402, -4.8647) (3.8671, -5.0916) (4.1005, -5.8112) (4.1005, -6.3233) knots 0 0 0 1 2 2 2
  spline S54 degree 2 poles (3.1053, -6.1742) (3.1053, -5.8468) (2.9951, -5.4254) (2.8947, -5.3087) knots 0 0 0 1 2 2 2
  spline S55 degree 2 poles (2.8947, -5.3087) (2.8266, -5.2212) (2.6515, -5.1467) (2.5511, -5.1467) knots 0 0 0 1 2 2 2
  spline S56 degree 2 poles (2.5511, -5.1467) (2.4603, -5.1467) (2.2917, -5.218) (2.2139, -5.3087) knots 0 0 0 1 2 2 2
  spline S57 degree 2 poles (2.2139, -5.3087) (2.1459, -5.3865) (2.0486, -5.688) (2.0486, -5.8663) knots 0 0 0 1 2 2 2
  spline S58 degree 2 poles (2.0486, -5.8663) (2.0486, -6.0608) (2.1491, -6.3104) (2.2334, -6.3849) knots 0 0 0 1 2 2 2
  spline S59 degree 2 poles (2.2334, -6.3849) (2.3209, -6.4595) (2.5381, -6.5178) (2.6742, -6.5178) knots 0 0 0 1 2 2 2
  spline S60 degree 2 poles (2.6742, -6.5178) (2.7877, -6.5178) (3.0243, -6.4562) (3.0989, -6.4238) knots 0 0 0 1 2 2 2
  spline S61 degree 2 poles (3.0989, -6.4238) (3.0989, -6.3946) (3.1053, -6.2844) (3.1053, -6.1742) knots 0 0 0 1 2 2 2
  point P0 (0, 12.5)
  point P1 (0, -12.5)
  point P2 (12.5, 0)
  point P3 (-12.5, 0)
  constraints: 4 midpoint, 4 point on circle, 2 other
emboss "Рельеф7" sketch "Эскиз4" operation cut depth 0.5 direction (0, 0, -1)
sketch "Эскиз5" plane through (14.2806, -14.2806, 2.2) normal (0, 0, 1) x (1, 0, 0)
  line L0 (-11, 11) -> (11, 11) construction
  line L1 (11, 11) -> (11, -11) construction
  line L2 (11, -11) -> (-11, -11) construction
  line L3 (-11, -11) -> (-11, 11) construction
  circle A0 centre (0, 0) radius 11 construction
  line L4 (-2.0891, 4.5454) -> (-4.731, 4.5454)
  line L5 (-4.731, 4.5454) -> (-4.731, 5.2423)
  line L6 (-4.731, 5.2423) -> (-3.8882, 5.2423)
  line L7 (-3.8882, 5.2423) -> (-3.8882, 7.359)
  line L8 (-3.8882, 7.359) -> (-4.731, 7.359)
  line L9 (-4.731, 7.359) -> (-4.731, 8.0105)
  spline S0 degree 2 poles (-4.731, 8.0105) (-4.5462, 8.0105) (-4.1799, 8.0592) (-4.0697, 8.111) knots 0 0 0 1 2 2 2
  spline S1 degree 2 poles (-4.0697, 8.111) (-3.9433, 8.1758) (-3.8006, 8.393) (-3.7877, 8.5551) knots 0 0 0 1 2 2 2
  line L10 (-3.7877, 8.5551) -> (-2.9125, 8.5551)
  line L11 (-2.9125, 8.5551) -> (-2.9125, 5.2423)
  line L12 (-2.9125, 5.2423) -> (-2.0891, 5.2423)
  line L13 (-2.0891, 5.2423) -> (-2.0891, 4.5454)
  spline S2 degree 2 poles (1.5413, 6.5454) (1.5413, 6.0267) (1.376, 5.2488) (1.1912, 4.9862) knots 0 0 0 1 2 2 2
  spline S3 degree 2 poles (1.1912, 4.9862) (1.0097, 4.7269) (0.423, 4.4611) (0.0016, 4.4611) knots 0 0 0 1 2 2 2
  spline S4 degree 2 poles (0.0016, 4.4611) (-0.423, 4.4611) (-1.0065, 4.7269) (-1.1912, 4.9927) knots 0 0 0 1 2 2 2
  spline S5 degree 2 poles (-1.1912, 4.9927) (-1.376, 5.2553) (-1.5413, 6.0267) (-1.5413, 6.5454) knots 0 0 0 1 2 2 2
  spline S6 degree 2 poles (-1.5413, 6.5454) (-1.5413, 7.077) (-1.376, 7.829) (-1.188, 8.1013) knots 0 0 0 1 2 2 2
  spline S7 degree 2 poles (-1.188, 8.1013) (-1, 8.3671) (-0.4068, 8.6264) (0.0016, 8.6264) knots 0 0 0 1 2 2 2
  spline S8 degree 2 poles (0.0016, 8.6264) (0.4327, 8.6264) (1.0097, 8.3541) (1.1945, 8.0851) knots 0 0 0 1 2 2 2
  spline S9 degree 2 poles (1.1945, 8.0851) (1.376, 7.8225) (1.5413, 7.0478) (1.5413, 6.5454) knots 0 0 0 1 2 2 2
  spline S10 degree 2 poles (0.5332, 6.5454) (0.5332, 7.2877) (0.2901, 7.8874) (0.0016, 7.8874) knots 0 0 0 1 2 2 2
  spline S11 degree 2 poles (0.0016, 7.8874) (-0.2869, 7.8874) (-0.5332, 7.2877) (-0.5332, 6.5421) knots 0 0 0 1 2 2 2
  spline S12 degree 2 poles (-0.5332, 6.5421) (-0.5332, 5.8096) (-0.2869, 5.2002) (0.0016, 5.2002) knots 0 0 0 1 2 2 2
  spline S13 degree 2 poles (0.0016, 5.2002) (0.2869, 5.2002) (0.5332, 5.8096) (0.5332, 6.5454) knots 0 0 0 1 2 2 2
  line L14 (4.1605, 5.6151) -> (4.1605, 5.0446)
  line L15 (4.1605, 5.0446) -> (3.0843, 5.0446)
  line L16 (3.0843, 5.0446) -> (3.0843, 4.5454)
  line L17 (3.0843, 4.5454) -> (2.0859, 4.5454)
  line L18 (2.0859, 4.5454) -> (2.0859, 5.0446)
  line L19 (2.0859, 5.0446) -> (1.8104, 5.0446)
  line L20 (1.8104, 5.0446) -> (1.8104, 5.6151)
  line L21 (1.8104, 5.6151) -> (2.0859, 5.6151)
  line L22 (2.0859, 5.6151) -> (2.0859, 6.0138)
  line L23 (2.0859, 6.0138) -> (1.8104, 6.0138)
  line L24 (1.8104, 6.0138) -> (1.8104, 6.7334)
  line L25 (1.8104, 6.7334) -> (2.0859, 6.7334)
  line L26 (2.0859, 6.7334) -> (2.0859, 8.5454)
  line L27 (2.0859, 8.5454) -> (3.6126, 8.5454)
  spline S14 degree 2 poles (3.6126, 8.5454) (3.9303, 8.5454) (4.4878, 8.4125) (4.8995, 8.1143) (5.1361, 7.6345) (5.1361, 7.2877) knots 0 0 0 1 2 3 4 4 4
  spline S15 degree 2 poles (5.1361, 7.2877) (5.1361, 6.9473) (4.893, 6.4643) (4.4749, 6.1564) (3.9109, 6.0138) (3.59, 6.0138) knots 0 0 0 1 2 3 4 4 4
  line L28 (3.59, 6.0138) -> (3.0843, 6.0138)
  line L29 (3.0843, 6.0138) -> (3.0843, 5.6151)
  line L30 (3.0843, 5.6151) -> (4.1605, 5.6151)
  spline S16 degree 2 poles (4.1053, 7.2617) (4.1053, 7.4562) (3.9335, 7.6734) (3.6677, 7.7836) (3.3501, 7.8096) (3.2042, 7.8096) knots 0 0 0 1 2 3 4 4 4
  line L31 (3.2042, 7.8096) -> (3.0843, 7.8096)
  line L32 (3.0843, 7.8096) -> (3.0843, 6.7334)
  line L33 (3.0843, 6.7334) -> (3.1264, 6.7334)
  spline S17 degree 2 poles (3.1264, 6.7334) (3.3241, 6.7334) (3.6775, 6.7561) (3.9465, 6.8598) (4.1053, 7.0705) (4.1053, 7.2617) knots 0 0 0 1 2 3 4 4 4
  line L34 (-0.1588, -2.0405) -> (-3.0989, -2.0405)
  line L35 (-3.0989, -2.0405) -> (-3.0989, -1.389)
  spline S18 degree 2 poles (-3.0989, -1.389) (-2.7261, -1.0908) (-2.1297, -0.5656) (-1.906, -0.329) knots 0 0 0 1 2 2 2
  spline S19 degree 2 poles (-1.906, -0.329) (-1.611, -0.0211) (-1.3485, 0.4489) (-1.3485, 0.6953) knots 0 0 0 1 2 2 2
  spline S20 degree 2 poles (-1.3485, 0.6953) (-1.3485, 0.9741) (-1.6823, 1.2723) (-1.9806, 1.2723) knots 0 0 0 1 2 2 2
  spline S21 degree 2 poles (-1.9806, 1.2723) (-2.1329, 1.2723) (-2.4052, 1.1977) (-2.5446, 1.1394) knots 0 0 0 1 2 2 2
  spline S22 degree 2 poles (-2.5446, 1.1394) (-2.6807, 1.0778) (-2.8752, 0.9481) (-2.9238, 0.9157) knots 0 0 0 1 2 2 2
  line L36 (-2.9238, 0.9157) -> (-3.0016, 0.9157)
  line L37 (-3.0016, 0.9157) -> (-3.0016, 1.7877)
  spline S23 degree 2 poles (-3.0016, 1.7877) (-2.8331, 1.8687) (-2.1135, 2.0373) (-1.7796, 2.0373) knots 0 0 0 1 2 2 2
  spline S24 degree 2 poles (-1.7796, 2.0373) (-1.0665, 2.0373) (-0.3339, 1.4019) (-0.3339, 0.8282) knots 0 0 0 1 2 2 2
  spline S25 degree 2 poles (-0.3339, 0.8282) (-0.3339, 0.4749) (-0.6677, -0.2058) (-1.0535, -0.5948) knots 0 0 0 1 2 2 2
  spline S26 degree 2 poles (-1.0535, -0.5948) (-1.2966, -0.8347) (-1.7536, -1.2075) (-1.8541, -1.2853) knots 0 0 0 1 2 2 2
  line L38 (-1.8541, -1.2853) -> (-0.1588, -1.2853)
  line L39 (-0.1588, -1.2853) -> (-0.1588, -2.0405)
  line L40 (3.3452, -2.0405) -> (0.4052, -2.0405)
  line L41 (0.4052, -2.0405) -> (0.4052, -1.389)
  spline S27 degree 2 poles (0.4052, -1.389) (0.778, -1.0908) (1.3744, -0.5656) (1.5981, -0.329) knots 0 0 0 1 2 2 2
  spline S28 degree 2 poles (1.5981, -0.329) (1.893, -0.0211) (2.1556, 0.4489) (2.1556, 0.6953) knots 0 0 0 1 2 2 2
  spline S29 degree 2 poles (2.1556, 0.6953) (2.1556, 0.9741) (1.8217, 1.2723) (1.5235, 1.2723) knots 0 0 0 1 2 2 2
  spline S30 degree 2 poles (1.5235, 1.2723) (1.3712, 1.2723) (1.0989, 1.1977) (0.9595, 1.1394) knots 0 0 0 1 2 2 2
  spline S31 degree 2 poles (0.9595, 1.1394) (0.8233, 1.0778) (0.6288, 0.9481) (0.5802, 0.9157) knots 0 0 0 1 2 2 2
  line L42 (0.5802, 0.9157) -> (0.5024, 0.9157)
  line L43 (0.5024, 0.9157) -> (0.5024, 1.7877)
  spline S32 degree 2 poles (0.5024, 1.7877) (0.671, 1.8687) (1.3906, 2.0373) (1.7245, 2.0373) knots 0 0 0 1 2 2 2
  spline S33 degree 2 poles (1.7245, 2.0373) (2.4376, 2.0373) (3.1702, 1.4019) (3.1702, 0.8282) knots 0 0 0 1 2 2 2
  spline S34 degree 2 poles (3.1702, 0.8282) (3.1702, 0.4749) (2.8363, -0.2058) (2.4506, -0.5948) knots 0 0 0 1 2 2 2
  spline S35 degree 2 poles (2.4506, -0.5948) (2.2075, -0.8347) (1.7504, -1.2075) (1.6499, -1.2853) knots 0 0 0 1 2 2 2
  line L44 (1.6499, -1.2853) -> (3.3452, -1.2853)
  line L45 (3.3452, -1.2853) -> (3.3452, -2.0405)
  line L46 (-1.0178, -8.6264) -> (-3.9579, -8.6264)
  line L47 (-3.9579, -8.6264) -> (-3.9579, -7.9749)
  spline S36 degree 2 poles (-3.9579, -7.9749) (-3.5851, -7.6767) (-2.9887, -7.1515) (-2.765, -6.9149) knots 0 0 0 1 2 2 2
  spline S37 degree 2 poles (-2.765, -6.9149) (-2.47, -6.607) (-2.2075, -6.1369) (-2.2075, -5.8906) knots 0 0 0 1 2 2 2
  spline S38 degree 2 poles (-2.2075, -5.8906) (-2.2075, -5.6118) (-2.5413, -5.3136) (-2.8395, -5.3136) knots 0 0 0 1 2 2 2
  spline S39 degree 2 poles (-2.8395, -5.3136) (-2.9919, -5.3136) (-3.2642, -5.3882) (-3.4036, -5.4465) knots 0 0 0 1 2 2 2
  spline S40 degree 2 poles (-3.4036, -5.4465) (-3.5397, -5.5081) (-3.7342, -5.6378) (-3.7828, -5.6702) knots 0 0 0 1 2 2 2
  line L48 (-3.7828, -5.6702) -> (-3.8606, -5.6702)
  line L49 (-3.8606, -5.6702) -> (-3.8606, -4.7982)
  spline S41 degree 2 poles (-3.8606, -4.7982) (-3.6921, -4.7172) (-2.9724, -4.5486) (-2.6386, -4.5486) knots 0 0 0 1 2 2 2
  spline S42 degree 2 poles (-2.6386, -4.5486) (-1.9254, -4.5486) (-1.1929, -5.1839) (-1.1929, -5.7577) knots 0 0 0 1 2 2 2
  spline S43 degree 2 poles (-1.1929, -5.7577) (-1.1929, -6.111) (-1.5267, -6.7917) (-1.9125, -7.1807) knots 0 0 0 1 2 2 2
  spline S44 degree 2 poles (-1.9125, -7.1807) (-2.1556, -7.4206) (-2.6126, -7.7933) (-2.7131, -7.8711) knots 0 0 0 1 2 2 2
  line L50 (-2.7131, -7.8711) -> (-1.0178, -7.8711)
  line L51 (-1.0178, -7.8711) -> (-1.0178, -8.6264)
  line L52 (0.4733, -8.6264) -> (-0.4765, -8.6264)
  line L53 (-0.4765, -8.6264) -> (-0.4765, -7.5697)
  line L54 (-0.4765, -7.5697) -> (0.4733, -7.5697)
  line L55 (0.4733, -7.5697) -> (0.4733, -8.6264)
  line L56 (4.2042, -8.6264) -> (1.2642, -8.6264)
  line L57 (1.2642, -8.6264) -> (1.2642, -7.9749)
  spline S45 degree 2 poles (1.2642, -7.9749) (1.637, -7.6767) (2.2334, -7.1515) (2.4571, -6.9149) knots 0 0 0 1 2 2 2
  spline S46 degree 2 poles (2.4571, -6.9149) (2.752, -6.607) (3.0146, -6.1369) (3.0146, -5.8906) knots 0 0 0 1 2 2 2
  spline S47 degree 2 poles (3.0146, -5.8906) (3.0146, -5.6118) (2.6807, -5.3136) (2.3825, -5.3136) knots 0 0 0 1 2 2 2
  spline S48 degree 2 poles (2.3825, -5.3136) (2.2301, -5.3136) (1.9579, -5.3882) (1.8185, -5.4465) knots 0 0 0 1 2 2 2
  spline S49 degree 2 poles (1.8185, -5.4465) (1.6823, -5.5081) (1.4878, -5.6378) (1.4392, -5.6702) knots 0 0 0 1 2 2 2
  line L58 (1.4392, -5.6702) -> (1.3614, -5.6702)
  line L59 (1.3614, -5.6702) -> (1.3614, -4.7982)
  spline S50 degree 2 poles (1.3614, -4.7982) (1.53, -4.7172) (2.2496, -4.5486) (2.5835, -4.5486) knots 0 0 0 1 2 2 2
  spline S51 degree 2 poles (2.5835, -4.5486) (3.2966, -4.5486) (4.0292, -5.1839) (4.0292, -5.7577) knots 0 0 0 1 2 2 2
  spline S52 degree 2 poles (4.0292, -5.7577) (4.0292, -6.111) (3.6953, -6.7917) (3.3096, -7.1807) knots 0 0 0 1 2 2 2
  spline S53 degree 2 poles (3.3096, -7.1807) (3.0665, -7.4206) (2.6094, -7.7933) (2.5089, -7.8711) knots 0 0 0 1 2 2 2
  line L60 (2.5089, -7.8711) -> (4.2042, -7.8711)
  line L61 (4.2042, -7.8711) -> (4.2042, -8.6264)
  point P0 (0, 11)
  point P1 (0, -11)
  point P2 (-11, 0)
  point P3 (11, 0)
  constraints: 4 midpoint, 4 point on circle, 2 other
emboss "Рельеф8" sketch "Эскиз5" operation cut depth 0.5 direction (0, 0, -1)
